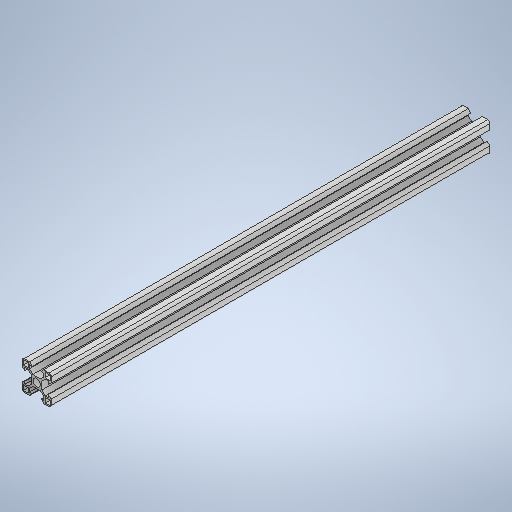
# Autodesk Inventor part: короткая палка
Saved by Autodesk Inventor 2025 (Build 290162000, 162)
## iProperties
Created: 2025-02-18
Part Number: короткая палка
Material: Типовые
Document SubType Name: Modeling
Designer: volko
Density: 1 g/cm^3
Appearance: По умолчанию
Author: volko
Autodesk Inventor part; units mm, degrees
ref_plane "YZ Plane" through (0, 0, 0) normal (1, 0, 0) x (0, 1, 0)
ref_plane "XZ Plane" through (0, 0, 0) normal (0, 1, 0) x (-1, 0, 0)
ref_plane "XY Plane" through (0, 0, 0) normal (0, 0, 1) x (1, 0, 0)
sketch "Эскиз1" plane through (0, 0, 0) normal (0, 0, 1) x (1, 0, 0)
  line L0 (-14.4349, 0) -> (14.4349, 0) projected
  line L1 (0, -14) -> (0, 14) projected
  line L2 (0, 0) -> (7.5, 7.5) construction
  circle A0 centre (7.5, 7.5) radius 1.65 construction
  line L3 (5.85, 9.15) -> (9.15, 9.15)
  line L4 (9.15, 9.15) -> (9.15, 5.85)
  line L5 (9.15, 5.85) -> (5.85, 5.85)
  line L6 (5.85, 5.85) -> (5.85, 9.15)
  line L7 (3.1, 8) -> (4.75, 10)
  line L8 (4.75, 10) -> (8.5, 10)
  line L9 (3.1, 8) -> (4.95, 8)
  line L10 (4.95, 8) -> (4.95, 5.7985)
  line L11 (4.95, 5.7985) -> (2.6515, 3.5)
  line L12 (0, 3.5) -> (2.6515, 3.5)
  circle A1 centre (0, 0) radius 2.5
  line L13 (8, 3.1) -> (10, 4.75)
  line L14 (10, 4.75) -> (10, 8.5)
  line L15 (8, 3.1) -> (8, 4.95)
  line L16 (8, 4.95) -> (5.7985, 4.95)
  line L17 (5.7985, 4.95) -> (3.5, 2.6515)
  line L18 (3.5, 0) -> (3.5, 2.6515)
  arc A2 (10, 8.5) -> (8.5, 10) centre (8.5, 8.5) ccw
  line L19 (0, 0) -> (-7.5, 7.5) construction
  circle A3 centre (-7.5, 7.5) radius 1.65 construction
  line L20 (-5.85, 9.15) -> (-9.15, 9.15)
  line L21 (-9.15, 9.15) -> (-9.15, 5.85)
  line L22 (-9.15, 5.85) -> (-5.85, 5.85)
  line L23 (-5.85, 5.85) -> (-5.85, 9.15)
  line L24 (-3.1, 8) -> (-4.75, 10)
  line L25 (-4.75, 10) -> (-8.5, 10)
  line L26 (-3.1, 8) -> (-4.95, 8)
  line L27 (-4.95, 8) -> (-4.95, 5.7985)
  line L28 (-4.95, 5.7985) -> (-2.6515, 3.5)
  line L29 (0, 3.5) -> (-2.6515, 3.5)
  line L30 (-3.5, 0) -> (-3.5, 2.6515)
  line L31 (-5.7985, 4.95) -> (-3.5, 2.6515)
  line L32 (-8, 4.95) -> (-5.7985, 4.95)
  line L33 (-8, 3.1) -> (-8, 4.95)
  line L34 (-8, 3.1) -> (-10, 4.75)
  line L35 (-10, 4.75) -> (-10, 8.5)
  arc A4 (-8.5, 10) -> (-10, 8.5) centre (-8.5, 8.5) ccw
  line L36 (0, 14) -> (0, -14)
  line L37 (0, 0) -> (7.5, -7.5) construction
  circle A5 centre (7.5, -7.5) radius 1.65 construction
  line L38 (5.85, -9.15) -> (9.15, -9.15)
  line L39 (9.15, -9.15) -> (9.15, -5.85)
  line L40 (9.15, -5.85) -> (5.85, -5.85)
  line L41 (5.85, -5.85) -> (5.85, -9.15)
  line L42 (3.1, -8) -> (4.75, -10)
  line L43 (4.75, -10) -> (8.5, -10)
  line L44 (3.1, -8) -> (4.95, -8)
  line L45 (4.95, -8) -> (4.95, -5.7985)
  line L46 (4.95, -5.7985) -> (2.6515, -3.5)
  line L47 (0, -3.5) -> (2.6515, -3.5)
  line L48 (3.5, 0) -> (3.5, -2.6515)
  line L49 (5.7985, -4.95) -> (3.5, -2.6515)
  line L50 (8, -4.95) -> (5.7985, -4.95)
  line L51 (8, -3.1) -> (8, -4.95)
  line L52 (8, -3.1) -> (10, -4.75)
  line L53 (10, -4.75) -> (10, -8.5)
  arc A6 (8.5, -10) -> (10, -8.5) centre (8.5, -8.5) ccw
  line L54 (0, 0) -> (-7.5, -7.5) construction
  line L55 (-4.95, -8) -> (-4.95, -5.7985)
  line L56 (-3.1, -8) -> (-4.95, -8)
  line L57 (-5.7985, -4.95) -> (-3.5, -2.6515)
  line L58 (-4.95, -5.7985) -> (-2.6515, -3.5)
  line L59 (-3.5, 0) -> (-3.5, -2.6515)
  line L60 (0, -3.5) -> (-2.6515, -3.5)
  circle A7 centre (-7.5, -7.5) radius 1.65 construction
  line L61 (-5.85, -5.85) -> (-5.85, -9.15)
  line L62 (-5.85, -9.15) -> (-9.15, -9.15)
  line L63 (-9.15, -9.15) -> (-9.15, -5.85)
  line L64 (-9.15, -5.85) -> (-5.85, -5.85)
  line L65 (-3.1, -8) -> (-4.75, -10)
  line L66 (-8, -4.95) -> (-5.7985, -4.95)
  line L67 (-8, -3.1) -> (-8, -4.95)
  line L68 (-8, -3.1) -> (-10, -4.75)
  line L69 (-4.75, -10) -> (-8.5, -10)
  line L70 (-10, -4.75) -> (-10, -8.5)
  arc A8 (-10, -8.5) -> (-8.5, -10) centre (-8.5, -8.5) ccw
  point P0 (7.5, 9.15)
  point P1 (7.5, 5.85)
  point P2 (9.15, 7.5)
  point P3 (-7.5, 9.15)
  point P4 (-7.5, 5.85)
  point P5 (-9.15, 7.5)
  point P6 (7.5, -9.15)
  point P7 (7.5, -5.85)
  point P8 (9.15, -7.5)
  point P9 (-7.5, -5.85)
  point P10 (-7.5, -9.15)
  point P11 (-9.15, -7.5)
  dimension "d0" = 45
  dimension "d1" = 3.3
  dimension "d2" = 1.5
  dimension "d3" = 1.2
  dimension "d4" = 5
  dimension "d5" = 6.5
  dimension "d6" = 15
  dimension "d7" = 20
  dimension "d8" = 9.9
  dimension "d9" = 9.5
  dimension "d10" = 6.2
  dimension "d11" = 2
  constraints: 138 end point, 76 symmetric about line, 20 point on circle, 9 centre point, 6 coincident, 3 equal length, 3 horizontal, 3 midpoint, 2 perpendicular, 2 point on line, 2 tangent, 1 parallel, 1 vertical, 6 other
  measures "d0" angle of L0 L2
  measures "d1" diameter of A0
  measures "d2" radius of A2
  measures "d3" distance between parallel lines of L17 L11
  measures "d4" diameter of A1
  measures "d5" distance between parallel lines of L25 L29
  measures "d6" distance of L2.end L19.end
  measures "d7" distance between parallel lines of L14 L35
  measures "d8" distance between parallel lines of L10 L27
  measures "d9" distance of L7.end L24.end
  measures "d10" distance of L7.start L26.start
  measures "d11" distance between parallel lines of L25 L26
extrude "Выдавливание1" add sketch "Эскиз1" along normal blind 300 contours A1 L1 L12 L11 L10 L9 L7 L8 A2 L14 L13 L15 L16 L17 L18 L0 | A1 L1 L0 | L0 L1 A1 | L0 L48 L49 L50 L51 L52 L53 A6 L43 L42 L44 L45 L46 L47 L1 A1 | L1 A1 L0 | L0 A1 L1 | A1 L0 L30 L31 L32 L33 L34 L35 A4 L25 L24 L26 L27 L28 L29 L1 | L1 L60 L58 L55 L56 L65 L69 A8 L70 L68 L67 L66 L57 L59 L0 A1 | L3 L4 L5 L6 | L23 L22 L21 L20 | L41 L40 L39 L38 | L61 L62 L63 L64
extrude "Выдавливание2" cut sketch "Эскиз1" along normal through all contours A1 L1 L0 | L0 L1 A1 | L1 A1 L0 | L0 A1 L1 | L3 L4 L5 L6 | L23 L22 L21 L20 | L41 L40 L39 L38 | L61 L62 L63 L64
